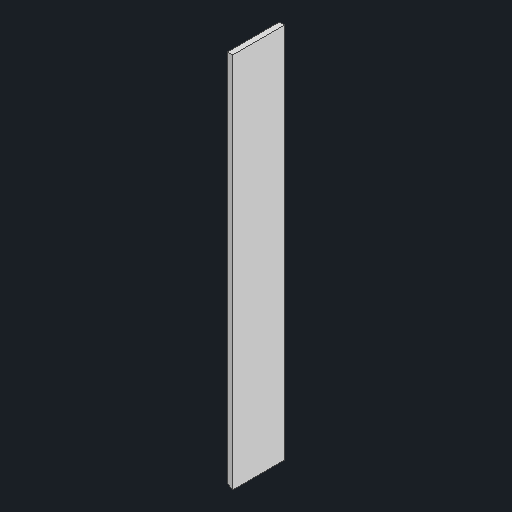
# Autodesk Inventor part: DMF 01 53 side part v2.1
Saved by Autodesk Inventor 2026.2 (Build 302298000, 298)
## iProperties
Created: 2024-05-05
Part Number: DMF 01 53 side part v2.1
Material: Generic
Document SubType Name: Modeling
Designer: pokla
Density: 1 g/cm^3
Appearance: Default
Author: pokla
Autodesk Inventor part; units mm, degrees
ref_plane "YZ Plane" through (0, 0, 0) normal (1, 0, 0) x (0, 1, 0)
ref_plane "XZ Plane" through (0, 0, 0) normal (0, 1, 0) x (-1, 0, 0)
ref_plane "XY Plane" through (0, 0, 0) normal (0, 0, 1) x (1, 0, 0)
sketch "Sketch1" plane through (0, 0, 0) normal (0, 0, 1) x (1, 0, 0)
  line L0 (0, 278.716) -> (197.082, 197.082) construction
  line L1 (197.082, 197.082) -> (278.716, 0) construction
  line L2 (278.716, 0) -> (197.082, -197.082) construction
  line L3 (197.082, -197.082) -> (0, -278.716) construction
  line L4 (0, -278.716) -> (-197.082, -197.082) construction
  line L5 (-197.082, -197.082) -> (-278.716, 0) construction
  line L6 (-278.716, 0) -> (-197.082, 197.082) construction
  line L7 (-197.082, 197.082) -> (0, 278.716) construction
  line L8 (-197.082, 197.082) -> (0, 278.716) construction
  line L9 (-461.6493, 774.8136) -> (-221.4406, 874.3113) construction
  line L10 (-98.541, 237.899) -> (-341.545, 824.5625) construction
  line L11 (-221.4406, 874.3113) -> (0, 874.3113) construction
  line L12 (0, 874.3113) -> (0, 278.716) construction
  line L13 (-461.6493, 774.8136) -> (-618.2315, 618.2315) construction
  line L14 (-618.2315, 618.2315) -> (-197.082, 197.082) construction
  line L15 (-5, 282.0569) -> (-195.9088, 202.9799) construction
  line L16 (-195.9088, 202.9799) -> (-611.1604, 618.2315) construction
  line L17 (-611.1604, 618.2315) -> (-458.817, 770.5748) construction
  line L18 (-458.817, 770.5748) -> (-220.4461, 869.3113) construction
  line L19 (-220.4461, 869.3113) -> (-5, 869.3113) construction
  line L20 (-5, 869.3113) -> (-5, 282.0569) construction
  line L21 (-13, 287.4023) -> (-194.0317, 212.4165) construction
  line L22 (-194.0317, 212.4165) -> (-599.8467, 618.2315) construction
  line L23 (-599.8467, 618.2315) -> (-454.2854, 763.7928) construction
  line L24 (-454.2854, 763.7928) -> (-218.8548, 861.3113) construction
  line L25 (-218.8548, 861.3113) -> (-13, 861.3113) construction
  line L26 (-13, 861.3113) -> (-13, 287.4023) construction
  line L27 (-13, 861.3113) -> (-5, 861.3113)
  line L28 (-5, 861.3113) -> (-5, 282.0569)
  line L29 (-5, 282.0569) -> (-13, 287.4023)
  line L30 (-13, 287.4023) -> (-13, 861.3113)
  point P0 (0, 0)
  point P1 (0, 0)
  point P2 (0, 0)
  dimension "d0" = 515
  dimension "d1" = 260
  dimension "d2" = 635
  dimension "d10" = 5
  dimension "d11" = 8
  constraints: 62 end point, 3 perpendicular, 2 coincident, 2 midpoint, 1 collinear, 1 horizontal, 1 parallel, 1 point on line, 1 symmetric about line, 1 vertical, 1 vertical alignment, 27 other
  measures "d0" distance between parallel lines of L5 L1
  measures "d1" distance of L13.start L11.start
  measures "d2" distance of L10.end L10.start
  measures "d10" distance between parallel lines of L12 L20
  measures "d11" distance between parallel lines of L20 L26
extrude "Extrusion1" add sketch "Sketch1" against normal blind 80
equation "\"d0\" = Барабан_размер_по_плоскостям"
equation "\"d1\" = Кассета_длина_грани"
equation "\"d2\" = Кассета_высота"
equation "\"Барабан_размер_по_плоскостям\" = 515"
equation "\"Кассета_длина_грани\" = 260"
equation "\"Кассета_высота\" = 635"
body "Solid1"
